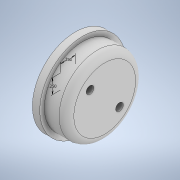
# Autodesk Inventor part: GL45 bottle cap insert
Saved by Autodesk Inventor 2020 (Build 240168000, 168)
## iProperties
Created: 2024-01-19
Part Number: GL45 bottle cap insert
Material: Generic
Document SubType Name: Modeling
Designer: Beaucage
Density: 1 g/cm^3
Appearance: Default
Author: Beaucage
Autodesk Inventor part; units mm, degrees
ref_plane "YZ Plane" through (0, 0, 0) normal (1, 0, 0) x (0, 1, 0)
ref_plane "XZ Plane" through (0, 0, 0) normal (0, 1, 0) x (-1, 0, 0)
ref_plane "XY Plane" through (0, 0, 0) normal (0, 0, 1) x (1, 0, 0)
sketch "Sketch1" plane through (0, 0, 0) normal (0, 1, 0) x (-1, 0, 0)
  line L0 (0, 0) -> (3.175, 0)
  line L1 (3.175, 0) -> (3.175, -18.5)
  line L2 (3.175, -18.5) -> (0, -18.5)
  line L3 (0, -18.5) -> (0, 0)
  line L4 (0, 0) -> (-9.525, 0)
  line L5 (-9.525, 0) -> (-9.525, -16.5)
  line L6 (-9.525, -16.5) -> (0, -16.5)
  line L7 (0, -16.5) -> (0, 0)
  line L8 (5.715, 0) -> (-12.065, 0) projected
  dimension "d0" = 3.175
  dimension "d1" = 18.5
  dimension "d2" = 9.525
  dimension "d3" = 16.5
  constraints: 16 end point, 4 parallel, 2 horizontal, 2 perpendicular
  measures "d0" distance of L1.end L2.end
  measures "d1" distance of L0.end L1.end
  measures "d2" distance of L6.end L5.end
  measures "d3" distance of L5.end L4.end
revolve "Revolution1" add sketch "Sketch1" angle 360 about axis through (-10, 0, 0) along (1, 0, 0)
sketch "Sketch2" plane through (-3.175, 0, 0) normal (-1, 0, 0) x (0, 0, 1)
  line L0 (0, 0) -> (6.35, 0)
  line L1 (6.35, 0) -> (6.35, 6.35)
  line L2 (6.35, 6.35) -> (0, 6.35)
  line L3 (0, 6.35) -> (0, 0)
  dimension "d5" = 6.35
  dimension "d6" = 6.35
  constraints: 8 end point, 2 parallel, 1 horizontal, 1 perpendicular
  measures "d5" distance of L2.end L1.end
  measures "d6" distance of L1.end L0.end
hole "Hole1" at (-3.175, 6.35, 6.35) direction (1, 0, 0) diameter 5.4102 depth 6.35
hole "Hole2" at (-3.175, 6.35, 6.35) direction (1, 0, 0) diameter 3.302 depth 12.7 tip angle 118
pattern_circular "Circular Pattern1" count 2 over 360 about axis through (-10, 0, 0) along (1, 0, 0) of "Hole1", "Hole2"
fillet "Fillet1" radius 3.175 1 edges at (9.525, 0, 16.5)
body "Solid1"
